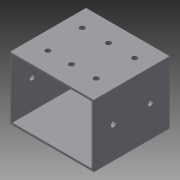
# Autodesk Inventor part: Box Base
Saved by Autodesk Inventor 2014 (Build 180170000, 170)
## iProperties
Created: 2014-05-19
Part Number: Box Base
Material: Generic
Document SubType Name: Modeling
Designer: lpluta-ehlers
Density: 1 g/cm^3
Appearance: Default
Author: lpluta-ehlers
Autodesk Inventor part; units mm, degrees
ref_plane "YZ Plane" through (0, 0, 0) normal (1, 0, 0) x (0, 1, 0)
ref_plane "XZ Plane" through (0, 0, 0) normal (0, 1, 0) x (-1, 0, 0)
ref_plane "XY Plane" through (0, 0, 0) normal (0, 0, 1) x (1, 0, 0)
sketch "Sketch1" plane through (0, 0, 0) normal (0, 1, 0) x (-1, 0, 0)
  line L0 (0, 0) -> (-203.2, 0)
  line L1 (-203.2, 0) -> (-203.2, -184.15)
  line L2 (-203.2, -184.15) -> (0, -184.15)
  line L3 (0, -184.15) -> (0, 0)
  dimension "blength" = 203.2
  dimension "bwidth" = 184.15
  constraints: 8 end point, 2 parallel, 1 horizontal, 1 perpendicular
  measures "blength" distance of L1.end L2.end
  measures "bwidth" distance of L0.end L1.end
extrude "Extrusion1" add sketch "Sketch1" along normal blind 152.4
shell "Shell1" thickness 6.35 removed faces 2 at (135.4667, 50.8, -184.15) at (67.7333, 50.8, 0)
fillet "Fillet1" radius 1.27 24 edges at (0, 152.4, -92.075) (101.6, 152.4, -184.15) (203.2, 152.4, -92.075) (101.6, 152.4, 0) (0, 76.2, -184.15) (6.35, 76.2, -184.15) (196.85, 76.2, -184.15) (101.6, 6.35, -184.15) (101.6, 146.05, -184.15) (203.2, 76.2, -184.15) (101.6, 0, -184.15) (6.35, 6.35, -92.075) (6.35, 146.05, -92.075) (196.85, 6.35, -92.075) (196.85, 146.05, -92.075) (6.35, 76.2, 0) (101.6, 6.35, 0) (196.85, 76.2, 0) (101.6, 146.05, 0) (0, 76.2, 0) (0, 0, -92.075) (101.6, 0, 0) (203.2, 76.2, 0) (203.2, 0, -92.075)
sketch "Sketch9" plane through (203.2, 1.27, -182.88) normal (1, 0, 0) x (0, 0, -1)
  line L0 (0, 0) -> (-181.61, 0) projected
  line L1 (0, 149.86) -> (0, 0) projected
  line L2 (-181.61, 0) -> (-181.61, 149.86) projected
  circle A0 centre (-135.5725, 76.2) radius 6.35
  circle A1 centre (-46.0375, 76.2) radius 6.35
  point P0 (-182.88, -1.27)
  dimension "csize" = 12.7
  dimension "d81" = 12.7
  dimension "d82" = 76.2
  dimension "d83" = 76.2
  dimension "d84" = 46.0375
  dimension "d85" = 46.0375
  constraints: 2 centre point
  measures "csize" diameter of A0
  measures "d81" diameter of A1
  measures "d82" distance from line of A1.centre L0
  measures "d83" distance from line of A0.centre L0
  measures "d84" distance from line of A0.centre L2
  measures "d85" distance from line of A1.centre L1
extrude "Extrusion6" cut sketch "Sketch9" against normal blind 6.35
sketch "Sketch10" plane through (0, 1.27, -1.27) normal (-1, 0, 0) x (0, 0, 1)
  line L0 (0, 0) -> (-181.61, 0) projected
  line L1 (0, 149.86) -> (0, 0) projected
  line L2 (-181.61, 0) -> (-181.61, 149.86) projected
  line L3 (0, 0) -> (-181.61, 0)
  line L4 (0, 149.86) -> (0, 0)
  line L5 (-181.61, 0) -> (-181.61, 149.86)
  circle A0 centre (-135.5725, 76.2) radius 6.35
  circle A1 centre (-46.0375, 76.2) radius 6.35
  point P0 (1.27, -1.27)
  point P1 (-182.88, -1.27)
  dimension "d106" = 12.7
  dimension "d107" = 12.7
  dimension "d108" = 46.0375
  dimension "d109" = 46.0375
  dimension "d110" = 76.2
  dimension "d111" = 76.2
  constraints: 6 end point, 2 centre point
  measures "d106" diameter of A0
  measures "d107" diameter of A1
  measures "d108" distance from line of A0.centre L2
  measures "d109" distance from line of A1.centre L1
  measures "d110" distance from line of A0.centre L0
  measures "d111" distance from line of A1.centre L0
sketch "Sketch11" plane through (0, 152.4, 0) normal (0, 1, 0) x (1, 0, 0)
  line L0 (201.93, 1.27) -> (1.27, 1.27) projected
  line L1 (201.93, 182.88) -> (201.93, 1.27) projected
  line L2 (1.27, 182.88) -> (201.93, 182.88) projected
  circle A0 centre (38.1, 136.8425) radius 6.35
  circle A1 centre (101.6, 136.8425) radius 6.35
  circle A2 centre (165.1, 136.8425) radius 6.35
  circle A3 centre (44.45, 47.3075) radius 6.35
  circle A4 centre (107.95, 47.3075) radius 6.35
  circle A5 centre (161.29, 47.3075) radius 6.35
  line L3 (1.27, 1.27) -> (1.27, 182.88) projected
  point P0 (0, 0)
  dimension "d112" = 12.7
  dimension "d113" = 12.7
  dimension "d114" = 12.7
  dimension "d115" = 46.0375
  dimension "d116" = 46.0375
  dimension "d117" = 46.0375
  dimension "d118" = 12.7
  dimension "d119" = 12.7
  dimension "d120" = 12.7
  dimension "d126" = 46.0375
  dimension "d127" = 46.0375
  dimension "d128" = 46.0375
  dimension "d134" = 40.64
  dimension "d135" = 106.68
  constraints: 6 centre point
  measures "d112" diameter of A0
  measures "d113" diameter of A1
  measures "d114" diameter of A2
  measures "d115" distance from line of A2.centre L2
  measures "d116" distance from line of A1.centre L2
  measures "d117" distance from line of A0.centre L2
  measures "d118" diameter of A3
  measures "d119" diameter of A4
  measures "d120" diameter of A5
  measures "d126" distance from line of A3.centre L0
  measures "d127" distance from line of L0 A4.centre
  measures "d128" distance from line of L0 A5.centre
  measures "d134" distance from line of A5.centre L1
  measures "d135" distance from line of A4.centre L3
extrude "Extrusion7" cut sketch "Sketch11" against normal blind 6.35 contours A0 | A1 | A2 | A3 | A4 | A5
extrude "Extrusion8" cut sketch "Sketch10" against normal blind 6.35
equation "\"d81\" = csize"
equation "\"d82\" = 0.5 * bheight"
equation "\"d83\" = 0.5 * bheight"
equation "\"d84\" = 0.25 * bwidth"
equation "\"d85\" = 0.25 * bwidth"
equation "\"d106\" = csize"
equation "\"d107\" = csize"
equation "\"d108\" = 0.25 * bwidth"
equation "\"d109\" = 0.25 * bwidth"
equation "\"d110\" = 0.5 * bheight"
equation "\"d111\" = 0.5 * bheight"
equation "\"d112\" = csize"
equation "\"d113\" = csize"
equation "\"d114\" = csize"
equation "\"d115\" = 0.25 * bwidth"
equation "\"d116\" = 0.25 * bwidth"
equation "\"d117\" = 0.25 * bwidth"
equation "\"d118\" = csize"
equation "\"d119\" = csize"
equation "\"d120\" = csize"
equation "\"d126\" = 0.25 * bwidth"
equation "\"d127\" = 0.25 * bwidth"
equation "\"d128\" = 0.25 * bwidth"
equation "\"d130\" = holeextrude"
equation "\"d132\" = holeextrude"
equation "\"topCircDistFromCntr\" = 0.2 * bwidth"
equation "\"bheight\" = 152.4"
equation "\"holeextrude\" = 6.35"
body "Solid1"
